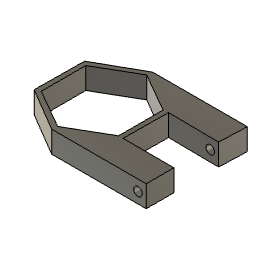
uchyt_hexagon (Autodesk Fusion 360 design; units mm, degrees)
Autodesk Fusion 360 part; units mm, degrees
sketch "Sketch1" plane through (0, 0, 0) normal (0, 0, 1) x (1, 0, 0)
  line L0 (-0.0194, 16.5) -> (-14.2991, 8.2332)
  line L1 (-14.2991, 8.2332) -> (-14.2797, -8.2668)
  line L2 (-14.2797, -8.2668) -> (0.0194, -16.5)
  line L3 (0.0194, -16.5) -> (14.2991, -8.2332)
  line L4 (14.2991, -8.2332) -> (14.2797, 8.2668)
  line L5 (14.2797, 8.2668) -> (-0.0194, 16.5)
  line L6 (0.2061, 18.4989) -> (-15.9174, 9.4279)
  line L7 (-15.9174, 9.4279) -> (-16.1235, -9.0709)
  line L8 (-16.1235, -9.0709) -> (-0.2061, -18.4989)
  line L9 (-0.2061, -18.4989) -> (15.9174, -9.4279)
  line L10 (15.9174, -9.4279) -> (16.1235, 9.0709)
  line L11 (16.1235, 9.0709) -> (0.2061, 18.4989)
  line L12 (0.2061, 18.4989) -> (35.2061, 18.5399)
  line L13 (35.2061, 18.5399) -> (34.8509, 8.2668)
  line L14 (34.8509, 8.2668) -> (16.1169, 8.4755)
  line L15 (0, 0) -> (14.2894, 0.0168)
  line L16 (-0.2061, -18.4989) -> (34.7939, -18.4989)
  line L17 (34.7939, -18.4989) -> (34.7939, -8.2199)
  line L18 (34.7939, -8.2199) -> (15.9309, -8.2199)
  dimension "d3" = 16.5
  dimension "d4" = 18.5
  dimension "d5" = 35
  dimension "d6" = 35
  dimension "d7" = 10.279
  constraint coincident L15.start origin
  constraint perpendicular L4 L12
  constraint coincident L10 L14.end
  constraint perpendicular L10 L14
  constraint midpoint L4 L15.end
  constraint horizontal L16
  constraint perpendicular L16 L17
  constraint coincident L10 L18.end
  constraint perpendicular L17 L18
  measures "d3" distance of L0.start L15.start
  measures "d4" distance of L6.start L15.start
  measures "d5" distance of L6.start L12.end
  measures "d6" distance of L8.end L16.end
  measures "d7" distance of L16.end L17.end
extrude "Extrude1" add sketch "Sketch1" along normal blind 8
sketch "Sketch2" plane through (-0.0217, 18.4986, 0) normal (-0.001173, 0.999999, 0) x (-0.999999, -0.001173, 0)
  line L0 (-35.2278, 0) -> (-0.2278, 0)
  line L1 (-0.2278, 0) -> (-0.2278, 8)
  line L2 (-0.2278, 8) -> (-35.2278, 8)
  line L3 (-35.2278, 8) -> (-35.2278, 0)
  line L4 (-35.2278, 4) -> (-31.7278, 4)
  circle A0 centre (-31.7278, 4) radius 1.6
  dimension "d10" = 3.5
  dimension "d11" = 3.2
  constraint midpoint L3 L4.start
  constraint perpendicular L3 L4
  constraint coincident L4.end A0.centre
  measures "d10" distance of L4.start L4.end
  measures "d11" diameter of A0
extrude "Extrude2" cut sketch "Sketch2" against normal blind 120 contours A0
